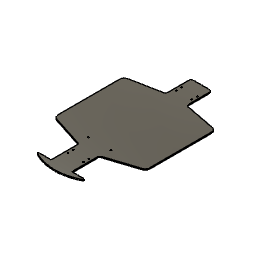
Bodenplatte v3 (Autodesk Fusion 360 design; units mm, degrees)
Autodesk Fusion 360 part; units mm, degrees
sketch "Skizze1" plane through (0, 0, 0) normal (0, 0, 1) x (1, 0, 0)
  line L0 (-100, 62.7184) -> (-100, -71.7499)
  line L1 (100, -71.7499) -> (100, 62.7184)
  line L2 (17.5, -150) -> (-17.5, -150)
  circle A0 centre (-17, -112) radius 1.55
  circle A1 centre (-17, -124) radius 1.55
  circle A2 centre (17, -112) radius 1.55
  circle A3 centre (17, -124) radius 1.55
  line L3 (-22.5, -145) -> (-22.5, -99.125)
  line L4 (22.5, -145) -> (22.5, -99.125)
  line L5 (-26.5499, -94.2162) -> (-91.9002, -81.5677)
  line L6 (26.5499, -94.2162) -> (91.9002, -81.5677)
  line L7 (-22.5, 150) -> (-22.5, 98.6408)
  line L8 (22.5, 150) -> (22.5, 98.6408)
  line L9 (-25.965, 93.8823) -> (-93.07, 72.2355)
  line L10 (25.965, 93.8823) -> (93.07, 72.2355)
  line L11 (-22.5, 150) -> (-22.5, 154)
  line L12 (-23.5, 155) -> (-50.0225, 155)
  line L13 (23.5, 155) -> (50.0225, 155)
  line L14 (22.5, 150) -> (22.5, 154)
  spline S0 degree 5 poles (-50.612, 156.8078) (-50.307, 157.0303) (-49.5138, 157.5768) (-48.0201, 158.4921) (-45.4608, 159.8491) (-41.335, 161.7172) (-36.0268, 163.7674) (-29.8884, 165.7539) (-23.0532, 167.5259) (-15.6772, 168.9326) (-7.9321, 169.8414) (0, 170.1573) (7.9321, 169.8414) (15.6772, 168.9326) (23.0532, 167.5259) (29.8884, 165.7539) (36.0268, 163.7674) (41.335, 161.7172) (45.4608, 159.8491) (48.0201, 158.4921) (49.5138, 157.5768) (50.307, 157.0303) (50.612, 156.8078) knots 0.06415 0.06415 0.06415 0.06415 0.06415 0.06415 0.1 0.15 0.2 0.25 0.3 0.35 0.4 0.45 0.5 0.55 0.6 0.65 0.7 0.75 0.8 0.85 0.9 0.93585 0.93585 0.93585 0.93585 0.93585 0.93585
  arc A4 (-50.612, 156.8078) -> (-50.0225, 155) centre (-50.0225, 156) ccw
  arc A5 (50.0225, 155) -> (50.612, 156.8078) centre (50.0225, 156) ccw
  arc A6 (-93.07, 72.2355) -> (-100, 62.7184) centre (-90, 62.7184) ccw
  arc A7 (100, 62.7184) -> (93.07, 72.2355) centre (90, 62.7184) ccw
  arc A8 (-100, -71.7499) -> (-91.9002, -81.5677) centre (-90, -71.7499) ccw
  arc A9 (91.9002, -81.5677) -> (100, -71.7499) centre (90, -71.7499) ccw
  arc A10 (-22.5, -99.125) -> (-26.5499, -94.2162) centre (-27.5, -99.125) ccw
  arc A11 (26.5499, -94.2162) -> (22.5, -99.125) centre (27.5, -99.125) ccw
  arc A12 (-22.5, -145) -> (-17.5, -150) centre (-17.5, -145) ccw
  arc A13 (17.5, -150) -> (22.5, -145) centre (17.5, -145) ccw
  arc A14 (-25.965, 93.8823) -> (-22.5, 98.6408) centre (-27.5, 98.6408) ccw
  arc A15 (22.5, 98.6408) -> (25.965, 93.8823) centre (27.5, 98.6408) ccw
  arc A16 (-22.5, 154) -> (-23.5, 155) centre (-23.5, 154) ccw
  arc A17 (23.5, 155) -> (22.5, 154) centre (23.5, 154) ccw
  circle A18 centre (-17, 124) radius 1.55
  circle A19 centre (-17, 112) radius 1.55
  circle A20 centre (17, 112) radius 1.55
  circle A21 centre (17, 124) radius 1.55
  circle A22 centre (-24.5, 72) radius 1.55
  circle A23 centre (24.5, 72) radius 1.55
  point P0 (22.5, -150)
  point P1 (-22.5, -95)
  point P2 (22.5, -95)
  point P3 (-22.5, 155)
  point P4 (-52.5, 155)
  point P5 (-45, 160)
  point P6 (0, 170)
  point P7 (45, 160)
  dimension "d15" = 3.1
  dimension "d16" = 3.1
  dimension "d17" = 3.1
  dimension "d18" = 3.1
  dimension "d20" = 55
  dimension "d25" = 30
  dimension "d27" = 1
  dimension "d28" = 1
  dimension "d29" = 10
  dimension "d30" = 10
  dimension "d31" = 10
  dimension "d32" = 10
  dimension "d33" = 5
  dimension "d34" = 5
  dimension "d35" = 5
  dimension "d36" = 5
  dimension "d37" = 5
  dimension "d38" = 5
  dimension "d39" = 1
  dimension "d40" = 1
  dimension "d41" = 3.1
  dimension "d42" = 3.1
  dimension "d43" = 3.1
  dimension "d44" = 3.1
  dimension "d50" = 3.1
  dimension "d51" = 3.1
  constraint parallel L0 L1
  constraint perpendicular L11 L12
  constraint coincident P4 L12
  constraint tangent L12 A4
  constraint tangent S0 A4
  constraint tangent S0 A5
  constraint tangent L13 A5
  constraint tangent L9 A6
  constraint tangent L0 A6
  constraint tangent L10 A7
  constraint tangent L1 A7
  constraint tangent L0 A8
  constraint tangent L5 A8
  constraint tangent L6 A9
  constraint tangent L1 A9
  constraint coincident P1 L5
  constraint coincident P1 L3
  constraint tangent L5 A10
  constraint tangent L3 A10
  constraint coincident P2 L6
  constraint coincident P2 L4
  constraint tangent L6 A11
  constraint tangent L4 A11
  constraint tangent L3 A12
  constraint coincident P0 L4
  constraint coincident P0 L2
  constraint tangent L4 A13
  constraint tangent L2 A13
  constraint tangent L7 A14
  constraint tangent L9 A14
  constraint tangent L8 A15
  constraint tangent L10 A15
  constraint coincident P3 L12
  constraint coincident P3 L11
  constraint tangent L12 A16
  constraint tangent L11 A16
  constraint tangent L13 A17
  constraint tangent L14 A17
  measures "d15" diameter of A0
  measures "d16" diameter of A1
  measures "d17" diameter of A2
  measures "d18" diameter of A3
  measures "d20" distance of P0 P2
  measures "d25" distance of P3 P4
  measures "d27" radius of A4
  measures "d28" radius of A5
  measures "d29" radius of A6
  measures "d30" radius of A7
  measures "d31" radius of A8
  measures "d32" radius of A9
  measures "d33" radius of A10
  measures "d34" radius of A11
  measures "d35" radius of A12
  measures "d36" radius of A13
  measures "d37" radius of A14
  measures "d38" radius of A15
  measures "d39" radius of A16
  measures "d40" radius of A17
  measures "d41" diameter of A18
  measures "d42" diameter of A19
  measures "d43" diameter of A20
  measures "d44" diameter of A21
  measures "d50" diameter of A22
  measures "d51" diameter of A23
extrude "Extrusion1" add sketch "Skizze1" along normal blind 2.5
move_body "Verschieben1" bodies 1 to x (-1, 0, 0) y (0, -1, 0) z (0, 0, 1) at (0, 0, 0)
named bodies: "Bodenplatte"
